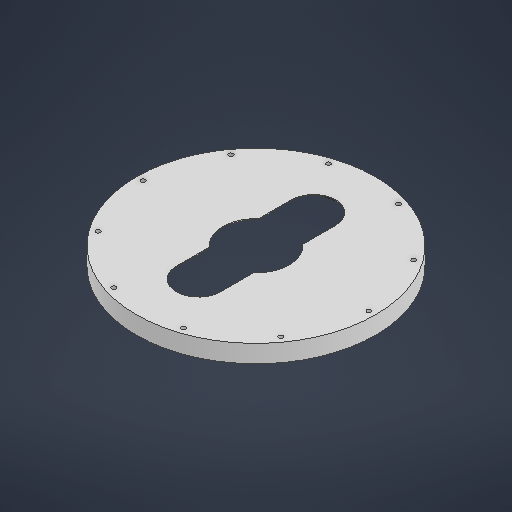
# Autodesk Inventor part: Cylinder Spacer Top
Saved by Autodesk Inventor 2025 (Build 290162000, 162)
## iProperties
Created: 2024-04-28
Part Number: Cylinder Spacer Top
Material: Generic
Document SubType Name: Modeling
Designer: Thienan Hoang
Density: 1 g/cm^3
Appearance: Default
Author: Thienan Hoang
Autodesk Inventor part; units mm, degrees
ref_plane "YZ Plane" through (0, 0, 0) normal (1, 0, 0) x (0, 1, 0)
ref_plane "XZ Plane" through (0, 0, 0) normal (0, 1, 0) x (-1, 0, 0)
ref_plane "XY Plane" through (0, 0, 0) normal (0, 0, 1) x (1, 0, 0)
sketch "Sketch1" plane through (0, 0, 0) normal (0, 1, 0) x (-1, 0, 0)
  circle A0 centre (0, 0) radius 135
  circle A1 centre (0, 0) radius 110
  dimension "d0" = 270
  dimension "d1" = 220
  constraints: 2 centre point, 2 coincident
  measures "d0" diameter of A0
  measures "d1" diameter of A1
extrude "Extrusion1" add sketch "Sketch1" along normal blind 55
sketch "Sketch2" plane through (0, 0, 0) normal (0, 0, 1) x (1, 0, 0)
  circle A0 centre (0, 5) radius 18
  line L0 (135, 0) -> (-135, 0) projected
  point P0 (0, 0)
  dimension "d4" = 36
  dimension "d5" = 5
  constraints: 1 centre point
  measures "d4" diameter of A0
  measures "d5" distance from line of L0 A0.centre
extrude "Extrusion2" cut sketch "Sketch2" against normal through all
sketch "Sketch3" plane through (0, 0, 0) normal (0, -1, 0) x (1, 0, 0)
  circle A0 centre (0, 0) radius 140
  constraints: 1 centre point, 1 coincident
extrude "Extrusion3" cut sketch "Sketch3" against normal blind 20
sketch "Sketch4" plane through (0, 20, 0) normal (0, -1, 0) x (1, 0, 0)
  line L0 (0, 0) -> (70, 0)
  line L1 (80, -100) -> (60, -100)
  line L2 (60, -100) -> (60, 100)
  line L3 (60, 100) -> (80, 100)
  line L4 (80, 100) -> (80, -100)
  line L5 (80, -100) -> (60, 100) construction
  line L6 (60, -100) -> (80, 100) construction
  dimension "d10" = 70
  dimension "d11" = 20
  dimension "d12" = 200
  constraints: 14 end point, 2 horizontal, 2 midpoint, 2 parallel, 1 perpendicular
  measures "d10" distance of L0.start L0.end
  measures "d11" distance of L2.end L3.end
  measures "d12" distance of L1.end L2.end
extrude "Extrusion4" cut sketch "Sketch4" against normal through all
sketch "Sketch5" plane through (0, 55, 0) normal (0, 1, 0) x (1, 0, 0)
  circle A0 centre (0, 0) radius 127.5
  circle A1 centre (127.5, 0) radius 2
  circle A2 centre (103.1497, 74.9426) radius 2
  circle A3 centre (39.3997, 121.2597) radius 2
  circle A4 centre (-39.3997, 121.2597) radius 2
  circle A5 centre (-103.1497, 74.9426) radius 2
  circle A6 centre (-127.5, 0) radius 2
  circle A7 centre (-103.1497, -74.9426) radius 2
  circle A8 centre (-39.3997, -121.2597) radius 2
  circle A9 centre (39.3997, -121.2597) radius 2
  circle A10 centre (103.1497, -74.9426) radius 2
  dimension "d15" = 255
  dimension "d16" = 4
  dimension "d19" = 360
  constraints: 10 centre point, 1 coincident, 1 horizontal alignment, 23 other
  measures "d16" diameter of A1
hole "Hole1" at (127.5, 55, 0) at (103.1497, 55, 74.9426) at (39.3997, 55, 121.2597) at (-39.3997, 55, 121.2597) at (-103.1497, 55, 74.9426) at (-127.5, 55, 0) at (-103.1497, 55, -74.9426) at (-39.3997, 55, -121.2597) at (39.3997, 55, -121.2597) at (103.1497, 55, -74.9426) direction (0, -1, 0) diameter 5 end through all
sketch "Sketch6" plane through (0, 55, 0) normal (0, 1, 0) x (1, 0, 0)
  circle A0 centre (0, 0) radius 140
  constraints: 1 centre point, 1 coincident
extrude "Extrusion5" cut sketch "Sketch6" against normal blind 15
sketch "Sketch7" plane through (0, 40, 0) normal (0, 1, 0) x (1, 0, 0)
  circle A0 centre (0, 0) radius 140
  line L0 (80, -100) -> (80, -75.4983) projected
  line L1 (80, -100) -> (80, -75.4983)
  line L2 (60, -100) -> (80, -100) projected
  line L3 (80, -100) -> (60, -100)
  line L4 (60, -100) -> (60, -92.1954)
  line L5 (60, 100) -> (60, 92.1954) projected
  line L6 (60, 92.1954) -> (60, 100)
  line L7 (60, 100) -> (80, 100)
  line L8 (80, 100) -> (80, 75.4983)
  arc A1 (80, -75.4983) -> (80, 75.4983) centre (0, 0) ccw
  arc A2 (60, 92.1954) -> (60, -92.1954) centre (0, 0) ccw
  arc A3 (-25, -65) -> (25, -65) centre (0, -65) ccw
  arc A4 (25, 65) -> (-25, 65) centre (0, 65) ccw
  arc A5 (25, -27.9508) -> (25, 27.9508) centre (0, 0) ccw
  arc A6 (-25, 27.9508) -> (-25, -27.9508) centre (0, 0) ccw
  line L9 (25, 65) -> (25, 27.9508)
  line L10 (25, -27.9508) -> (25, -65)
  line L11 (-25, -65) -> (-25, -27.9508)
  line L12 (-25, 27.9508) -> (-25, 65)
  constraints: 20 end point, 12 point on circle, 7 centre point, 7 equal length, 3 perpendicular, 2 coincident
extrude "Extrusion6" add sketch "Sketch7" against normal blind 1 contours L2 L4 A2 L5 L7 L8 A1 L0
sketch "Sketch8" plane through (0, 39, 0) normal (0, -1, 0) x (1, 0, 0)
  line L0 (80, -75.4983) -> (80, -100) projected
  line L1 (80, -100) -> (60, -100)
  line L2 (60, -100) -> (60, 100)
  line L3 (60, 100) -> (80, 100)
  line L4 (80, 100) -> (80, 75.4983)
  line L5 (80, -75.4983) -> (80, -100)
  arc A0 (80, -75.4983) -> (80, 75.4983) centre (0, 0) ccw
  arc A1 (60, 92.1954) -> (60, -92.1954) centre (0, 0) ccw
  constraints: 10 end point, 4 point on circle, 3 parallel, 2 centre point, 2 point on line, 1 coincident, 1 horizontal, 1 perpendicular
extrude "Extrusion7" add sketch "Sketch8" along normal blind 14 contours L0 L1 L2 L3 L4 A0
body "Solid1"
